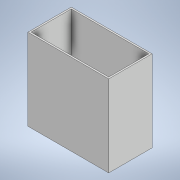
# Autodesk Inventor part: MagicBox
Saved by Autodesk Inventor 2020 (Build 240168000, 168)
## iProperties
Created: 2020-05-20
Part Number: MagicBox
Material: Generic
Document SubType Name: Modeling
Designer: user
Density: 1 g/cm^3
Appearance: Default
Author: user
## iProperties of the stored document _3DPrint.ipt
Created: 2020-05-20
Part Number: _3DPrint
Material: Generic
Document SubType Name: Modeling
Designer: user
Density: 1 g/cm^3
Appearance: Default
Author: user
Autodesk Inventor part; units mm, degrees
ref_plane "YZ Plane" through (0, 0, 0) normal (1, 0, 0) x (0, 1, 0)
ref_plane "XZ Plane" through (0, 0, 0) normal (0, 1, 0) x (-1, 0, 0)
ref_plane "XY Plane" through (0, 0, 0) normal (0, 0, 1) x (1, 0, 0)
sketch "Sketch1" plane through (0, 0, 0) normal (0, 1, 0) x (-1, 0, 0)
  line L0 (4.0152, 32.5375) -> (-70.4848, 32.5375)
  line L1 (-70.4848, 32.5375) -> (-70.4848, -7.4625)
  line L2 (-70.4848, -7.4625) -> (4.0152, -7.4625)
  line L3 (4.0152, -7.4625) -> (4.0152, 32.5375)
  point P0 (0, 0)
  dimension "d0" = 74.5
  dimension "d1" = 40
  constraints: 8 end point, 2 parallel, 1 horizontal, 1 perpendicular
  measures "d0" distance of L2.end L1.end
  measures "d1" distance of L1.end L0.end
extrude "Extrusion1" add sketch "Sketch1" along normal blind 75
sketch "Sketch2" plane through (0, 75, 0) normal (0, 1, 0) x (1, 0, 0)
  line L0 (-2.5152, -31.0375) -> (68.9848, -31.0375)
  line L1 (68.9848, -31.0375) -> (68.9848, 5.9625)
  line L2 (68.9848, 5.9625) -> (-2.5152, 5.9625)
  line L3 (-2.5152, 5.9625) -> (-2.5152, -31.0375)
  line L4 (-4.0152, 7.4625) -> (-4.0152, -32.5375) projected
  line L5 (70.4848, 7.4625) -> (-4.0152, 7.4625) projected
  line L6 (-4.0152, -32.5375) -> (70.4848, -32.5375) projected
  line L7 (70.4848, -32.5375) -> (70.4848, 7.4625) projected
  point P0 (0, 0)
  dimension "d4" = 1.5
  dimension "d5" = 1.5
  dimension "d6" = 1.5
  dimension "d7" = 1.5
  constraints: 8 end point, 2 parallel, 1 horizontal, 1 perpendicular
  measures "d4" distance between parallel lines of L3 L4
  measures "d5" distance between parallel lines of L5 L2
  measures "d6" distance between parallel lines of L6 L0
  measures "d7" distance between parallel lines of L7 L1
extrude "Extrusion2" cut sketch "Sketch2" against normal blind 73.5 contours L3 L2 L1 L0
equation "\"d5\" = d4"
equation "\"d6\" = d4"
equation "\"d7\" = d4"
body "Solid1"
